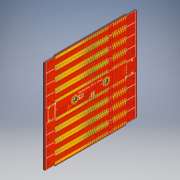
# Autodesk Inventor part: Backplane_PCB
Saved by Autodesk Inventor 2018 (Build 220112000, 112)
## iProperties
Created: 2018-10-18
Part Number: Backplane_PCB
Material: Epoxy Resin
Document SubType Name: Modeling
Designer: Bradley
Density: 1.14 g/cm^3
Appearance: Smooth - Dark Gray
Author: Bradley
Autodesk Inventor part; units mm, degrees
ref_plane "YZ Plane" through (0, 0, 0) normal (1, 0, 0) x (0, 1, 0)
ref_plane "XZ Plane" through (0, 0, 0) normal (0, 1, 0) x (-1, 0, 0)
ref_plane "XY Plane" through (0, 0, 0) normal (0, 0, 1) x (1, 0, 0)
sketch "Sketch1" plane through (0, 0, 0) normal (1, 0, 0) x (0, 1, 0)
  line L0 (-41.4, -43) -> (41.4, -43)
  line L1 (41.4, -43) -> (41.4, 43)
  line L2 (41.4, 43) -> (-41.4, 43)
  line L3 (-41.4, 43) -> (-41.4, -43)
  line L4 (-41.4, -43) -> (41.4, 43) construction
  line L5 (41.4, -43) -> (-41.4, 43) construction
  point P0 (0, 0)
  dimension "d0" = 86
  dimension "d1" = 82.8
  constraints: 12 end point, 2 midpoint, 2 parallel, 1 horizontal, 1 perpendicular
  measures "d0" distance of L2.end L0.start
  measures "d1" distance of L1.end L2.end
extrude "Extrusion1" add sketch "Sketch1" along normal mid plane 1
sketch "Sketch9" plane through (0.5, 0, 0) normal (1, 0, 0) x (0, 0, -1)
  line L0 (43, -41.4) -> (43, 41.4) projected
  line L1 (43, 41.4) -> (-43, 41.4) projected
  line L2 (-43, 41.4) -> (-43, -41.4) projected
  line L3 (-43, -41.4) -> (43, -41.4) projected
  line L4 (45, 36.5) -> (-45, 36.5) construction
  line L5 (-45, 36.5) -> (-45, -36.5) construction
  line L6 (-45, -36.5) -> (45, -36.5) construction
  line L7 (45, -36.5) -> (45, 36.5) construction
  line L8 (45, 36.5) -> (-45, -36.5) construction
  line L9 (-45, 36.5) -> (45, -36.5) construction
  circle A0 centre (-45, -36.5) radius 3 construction
  line L10 (-41.9, -41.4) -> (-41.9, -32)
  line L11 (-41.9, -32) -> (-43, -32)
  line L12 (-43, 41.4) -> (-43, -41.4) projected
  line L13 (-41.9, 41.4) -> (-41.9, 32)
  line L14 (-41.9, 32) -> (-43, 32)
  line L15 (43, 41.4) -> (-43, 41.4) projected
  line L16 (41.9, 41.4) -> (41.9, 32)
  line L17 (41.9, 32) -> (43, 32)
  line L18 (41.9, -41.4) -> (41.9, -32)
  line L19 (41.9, -32) -> (43, -32)
  point P0 (0, 0)
  dimension "d57" = 90
  dimension "d58" = 73
  dimension "d59" = 6
  dimension "d60" = 1.1
  dimension "d61" = 32
  constraints: 28 end point, 8 point on line, 6 collinear, 6 perpendicular, 3 vertical, 2 midpoint, 2 parallel, 1 centre point, 1 coincident, 1 horizontal
  measures "d57" distance of L6.end L5.end
  measures "d58" distance of L5.end L4.end
  measures "d59" diameter of A0
  measures "d60" distance between parallel lines of L10 L2
  measures "d61" distance from line of point (0, 0) L11
extrude "Extrusion2" cut sketch "Sketch9" against normal through all contours L3 L18 L19 L0 | L17 L16 L1 L0 | L3 L2 L11 L10 | L13 L14 L2 L1
fillet "Fillet1" radius 0.5 12 edges at (0, -41.4, -41.9) (0, -32, -41.9) (0, -32, -43) (0, 41.4, -41.9) (0, 32, -41.9) (0, 32, -43) (0, 41.4, 41.9) (0, 32, 43) (0, 32, 41.9) (0, -32, 43) (0, -32, 41.9) (0, -41.4, 41.9)
sketch "Sketch7" plane through (0.5, 0, 0) normal (1, 0, 0) x (0, 0, -1)
  line L0 (43, -31.5) -> (43, 31.5) projected
  line L1 (41.4, 41.4) -> (-41.4, 41.4) projected
  line L2 (-43, 31.5) -> (-43, -31.5) projected
  line L3 (-41.4, -41.4) -> (41.4, -41.4) projected
  line L4 (-43, -41.4) -> (43, -41.4) projected
  line L5 (43, 41.4) -> (-43, 41.4) projected
  arc A0 (-41.9, -40.9) -> (-41.4, -41.4) centre (-41.4, -40.9) ccw projected
  arc A1 (41.4, -41.4) -> (41.9, -40.9) centre (41.4, -40.9) ccw projected
  line L6 (41.9, -40.9) -> (41.9, -32.5) projected
  arc A2 (42.4, -32) -> (41.9, -32.5) centre (42.4, -32.5) ccw projected
  line L7 (42.4, -32) -> (42.5, -32) projected
  arc A3 (42.5, -32) -> (43, -31.5) centre (42.5, -31.5) ccw projected
  arc A4 (43, 31.5) -> (42.5, 32) centre (42.5, 31.5) ccw projected
  line L8 (42.5, 32) -> (42.4, 32) projected
  arc A5 (41.9, 32.5) -> (42.4, 32) centre (42.4, 32.5) ccw projected
  line L9 (41.9, 32.5) -> (41.9, 40.9) projected
  arc A6 (41.9, 40.9) -> (41.4, 41.4) centre (41.4, 40.9) ccw projected
  arc A7 (-41.4, 41.4) -> (-41.9, 40.9) centre (-41.4, 40.9) ccw projected
  line L10 (-41.9, 40.9) -> (-41.9, 32.5) projected
  arc A8 (-42.4, 32) -> (-41.9, 32.5) centre (-42.4, 32.5) ccw projected
  line L11 (-42.4, 32) -> (-42.5, 32) projected
  arc A9 (-42.5, 32) -> (-43, 31.5) centre (-42.5, 31.5) ccw projected
  arc A10 (-43, -31.5) -> (-42.5, -32) centre (-42.5, -31.5) ccw projected
  line L12 (-42.5, -32) -> (-42.4, -32) projected
  arc A11 (-41.9, -32.5) -> (-42.4, -32) centre (-42.4, -32.5) ccw projected
  line L13 (-41.9, -32.5) -> (-41.9, -40.9) projected
  line L14 (-43.0019, -41.4) -> (-43.0019, 41.4) construction
  line L15 (-43.0019, 41.4) -> (43.0019, 41.4) construction
  line L16 (43.0019, 41.4) -> (43.0019, -41.4) construction
  line L17 (43.0019, -41.4) -> (-43.0019, -41.4) construction
  point P0 (0, 0)
  point P1 (0, 41.4)
  point P2 (0, 41.4)
  constraints: 3 midpoint, 2 collinear, 2 other
decal "Decal1"
sketch "Sketch8" plane through (-0.5, 0, 0) normal (-1, 0, 0) x (0, 0, 1)
  line L0 (-43, 31.5) -> (-43, -31.5) projected
  line L1 (-41.4, -41.4) -> (41.4, -41.4) projected
  line L2 (43, -31.5) -> (43, 31.5) projected
  line L3 (41.4, 41.4) -> (-41.4, 41.4) projected
  line L4 (43, 41.4) -> (-43, 41.4) projected
  line L5 (-43, -41.4) -> (43, -41.4) projected
  arc A0 (41.4, -41.4) -> (41.9, -40.9) centre (41.4, -40.9) ccw projected
  line L6 (41.9, -40.9) -> (41.9, -32.5) projected
  arc A1 (42.4, -32) -> (41.9, -32.5) centre (42.4, -32.5) ccw projected
  line L7 (42.4, -32) -> (42.5, -32) projected
  arc A2 (42.5, -32) -> (43, -31.5) centre (42.5, -31.5) ccw projected
  arc A3 (43, 31.5) -> (42.5, 32) centre (42.5, 31.5) ccw projected
  line L8 (42.5, 32) -> (42.4, 32) projected
  arc A4 (41.9, 32.5) -> (42.4, 32) centre (42.4, 32.5) ccw projected
  line L9 (41.9, 32.5) -> (41.9, 40.9) projected
  arc A5 (41.9, 40.9) -> (41.4, 41.4) centre (41.4, 40.9) ccw projected
  arc A6 (-41.4, 41.4) -> (-41.9, 40.9) centre (-41.4, 40.9) ccw projected
  line L10 (-41.9, 40.9) -> (-41.9, 32.5) projected
  arc A7 (-42.4, 32) -> (-41.9, 32.5) centre (-42.4, 32.5) ccw projected
  line L11 (-42.4, 32) -> (-42.5, 32) projected
  arc A8 (-42.5, 32) -> (-43, 31.5) centre (-42.5, 31.5) ccw projected
  arc A9 (-43, -31.5) -> (-42.5, -32) centre (-42.5, -31.5) ccw projected
  line L12 (-42.5, -32) -> (-42.4, -32) projected
  arc A10 (-41.9, -32.5) -> (-42.4, -32) centre (-42.4, -32.5) ccw projected
  line L13 (-41.9, -32.5) -> (-41.9, -40.9) projected
  arc A11 (-41.9, -40.9) -> (-41.4, -41.4) centre (-41.4, -40.9) ccw projected
  line L14 (43.0019, 41.4) -> (43.0019, -41.4) construction
  line L15 (43.0019, -41.4) -> (-43.0019, -41.4) construction
  line L16 (-43.0019, -41.4) -> (-43.0019, 41.4) construction
  line L17 (-43.0019, 41.4) -> (43.0019, 41.4) construction
  point P0 (0, 0)
  point P1 (0, -41.4)
  point P2 (0, -41.4)
  constraints: 3 midpoint, 2 collinear, 2 other
decal "Decal2"
sketch "Sketch2" plane through (0.5, 0, 0) normal (1, 0, 0) x (0, 0, -1)
  line L0 (0, -14) -> (0, 14) construction
  point P0 (0, 0)
  point P1 (0, 0)
  dimension "d7" = 28
  constraints: 3 coincident, 2 end point, 1 midpoint, 1 vertical
  measures "d7" distance of L0.start L0.end
hole "Hole1" at (0.5, -14, 0) at (0.5, 14, 0) direction (-1, 0, 0) diameter 3.3 end through all
sketch "Sketch3" plane through (0.5, 0, 0) normal (1, 0, 0) x (0, 0, -1)
  point P0 (0, 0)
  point P1 (-37.5, 38.3)
  point P2 (-28.5, 38.3)
  point P3 (-19.5, 38.3)
  point P4 (-10.5, 38.3)
  point P5 (10.5, 38.3)
  point P6 (19.5, 38.3)
  point P7 (28.5, 38.3)
  point P8 (37.5, 38.3)
  constraints: 8 other
hole "Hole2" at (0.5, 38.3, 37.5) at (0.5, 38.3, 28.5) at (0.5, 38.3, 19.5) at (0.5, 38.3, 10.5) at (0.5, 38.3, -10.5) at (0.5, 38.3, -19.5) at (0.5, 38.3, -28.5) at (0.5, 38.3, -37.5) direction (-1, 0, 0) diameter 1.05 end through all
sketch "Sketch4" plane through (0.5, 0, 0) normal (1, 0, 0) x (0, 0, -1)
  point P0 (0, 0)
  point P1 (-37.5, -38.3)
  point P2 (-28.5, -38.3)
  point P3 (-19.5, -38.3)
  point P4 (-10.5, -38.3)
  point P5 (10.5, -38.3)
  point P6 (19.5, -38.3)
  point P7 (28.5, -38.3)
  point P8 (37.5, -38.3)
  constraints: 8 other
hole "Hole3" at (0.5, -38.3, 37.5) at (0.5, -38.3, 28.5) at (0.5, -38.3, 19.5) at (0.5, -38.3, 10.5) at (0.5, -38.3, -10.5) at (0.5, -38.3, -19.5) at (0.5, -38.3, -28.5) at (0.5, -38.3, -37.5) direction (-1, 0, 0) diameter 1.45 end through all
sketch "Sketch5" plane through (0.5, 0, 0) normal (1, 0, 0) x (0, 0, -1)
  point P0 (0, 0)
  point P1 (0, -16.3)
  point P2 (0, -11.7)
  point P3 (1.626, -12.374)
  point P4 (2.3, -14)
  point P5 (1.626, -15.626)
  point P6 (-2.3, -14)
  point P7 (-1.626, -15.626)
  point P8 (-1.626, -12.374)
  point P9 (-1.626, 15.626)
  point P10 (0, 11.7)
  point P11 (0, 16.3)
  point P12 (1.626, 15.626)
  point P13 (2.3, 14)
  point P14 (1.626, 12.374)
  point P15 (-2.3, 14)
  point P16 (-1.626, 12.374)
  constraints: 16 other
hole "Hole4" at (0.5, -16.3, 0) at (0.5, -11.7, 0) at (0.5, -12.374, -1.626) at (0.5, -14, -2.3) at (0.5, -15.626, -1.626) at (0.5, -14, 2.3) at (0.5, -15.626, 1.626) at (0.5, -12.374, 1.626) at (0.5, 15.626, 1.626) at (0.5, 11.7, 0) at (0.5, 16.3, 0) at (0.5, 15.626, -1.626) at (0.5, 14, -2.3) at (0.5, 12.374, -1.626) at (0.5, 14, 2.3) at (0.5, 12.374, 1.626) direction (-1, 0, 0) diameter 0.45 end through all
sketch "Sketch10" plane through (0.5, 0, 0) normal (1, 0, 0) x (0, 0, -1)
  point P0 (0, 0)
  point P1 (17.575, -9.45)
  point P2 (8.575, -9.45)
  point P3 (-12.425, -9.45)
  point P4 (-21.425, -9.45)
  point P5 (-30.425, -9.45)
  point P6 (-39.425, -9.45)
  point P7 (35.575, -10.65)
  point P8 (26.575, -10.65)
  point P9 (17.575, -10.65)
  point P10 (8.575, -10.65)
  point P11 (-12.425, -10.65)
  point P12 (-21.425, -10.65)
  point P13 (-30.425, -10.65)
  point P14 (-39.425, -10.65)
  point P15 (35.575, -16.65)
  point P16 (26.575, -16.65)
  point P17 (17.575, -16.65)
  point P18 (8.575, -16.65)
  point P19 (-12.425, -16.65)
  point P20 (-21.425, -16.65)
  point P21 (-30.425, -16.65)
  point P22 (-39.425, -16.65)
  point P23 (35.575, -17.85)
  point P24 (26.575, -17.85)
  point P25 (17.575, -17.85)
  point P26 (8.575, -17.85)
  point P27 (-12.425, -17.85)
  point P28 (-21.425, -17.85)
  point P29 (-30.425, -17.85)
  point P30 (-39.425, -17.85)
  point P31 (35.575, -19.05)
  point P32 (26.575, -19.05)
  point P33 (17.575, -19.05)
  point P34 (8.575, -19.05)
  point P35 (-12.425, -19.05)
  point P36 (-21.425, -19.05)
  point P37 (-30.425, -19.05)
  point P38 (-39.425, -19.05)
  point P39 (35.575, -21.45)
  point P40 (26.575, -21.45)
  point P41 (17.575, -21.45)
  point P42 (8.575, -21.45)
  point P43 (-12.425, -21.45)
  point P44 (-21.425, -21.45)
  point P45 (-30.425, -21.45)
  point P46 (-39.425, -21.45)
  point P47 (35.575, -22.65)
  point P48 (26.575, -22.65)
  point P49 (17.575, -22.65)
  point P50 (8.575, -22.65)
  point P51 (-12.425, -22.65)
  point P52 (-21.425, -22.65)
  point P53 (-30.425, -22.65)
  point P54 (-39.425, -22.65)
  point P55 (35.575, -11.85)
  point P56 (26.575, -11.85)
  point P57 (17.575, -11.85)
  point P58 (8.575, -11.85)
  point P59 (-12.425, -11.85)
  point P60 (-21.425, -11.85)
  point P61 (-30.425, -11.85)
  point P62 (-39.425, -11.85)
  point P63 (35.575, -13.05)
  point P64 (26.575, -13.05)
  point P65 (17.575, -13.05)
  point P66 (8.575, -13.05)
  point P67 (-12.425, -13.05)
  point P68 (-21.425, -13.05)
  point P69 (-30.425, -13.05)
  point P70 (-39.425, -13.05)
  point P71 (35.575, -14.25)
  point P72 (26.575, -14.25)
  point P73 (17.575, -14.25)
  point P74 (8.575, -14.25)
  point P75 (-12.425, -14.25)
  point P76 (-21.425, -14.25)
  point P77 (-30.425, -14.25)
  point P78 (-39.425, -14.25)
  point P79 (35.575, -15.45)
  point P80 (26.575, -15.45)
  point P81 (17.575, -15.45)
  point P82 (8.575, -15.45)
  point P83 (-12.425, -15.45)
  point P84 (-21.425, -15.45)
  point P85 (-30.425, -15.45)
  point P86 (-39.425, -15.45)
  point P87 (35.575, 3.75)
  point P88 (26.575, 3.75)
  point P89 (17.575, 3.75)
  point P90 (8.575, 3.75)
  point P91 (-12.425, 3.75)
  point P92 (-21.425, 3.75)
  point P93 (-30.425, 3.75)
  point P94 (-39.425, 3.75)
  point P95 (35.575, 2.55)
  point P96 (26.575, 2.55)
  point P97 (17.575, 2.55)
  point P98 (8.575, 2.55)
  point P99 (-12.425, 2.55)
  point P100 (-21.425, 2.55)
  point P101 (-30.425, 2.55)
  point P102 (-39.425, 2.55)
  point P103 (35.575, 1.35)
  point P104 (26.575, 1.35)
  point P105 (17.575, 1.35)
  point P106 (8.575, 1.35)
  point P107 (-12.425, 1.35)
  point P108 (-21.425, 1.35)
  point P109 (-30.425, 1.35)
  point P110 (-39.425, 1.35)
  point P111 (35.575, -1.05)
  point P112 (26.575, -1.05)
  point P113 (17.575, -1.05)
  point P114 (8.575, -1.05)
  point P115 (-12.425, -1.05)
  point P116 (-21.425, -1.05)
  point P117 (-30.425, -1.05)
  point P118 (-39.425, -1.05)
  point P119 (35.575, -2.25)
  point P120 (26.575, -2.25)
  point P121 (17.575, -2.25)
  point P122 (8.575, -2.25)
  point P123 (-12.425, -2.25)
  point P124 (-21.425, -2.25)
  point P125 (-30.425, -2.25)
  point P126 (-39.425, -2.25)
  point P127 (35.575, -3.45)
  point P128 (26.575, -3.45)
  point P129 (17.575, -3.45)
  point P130 (8.575, -3.45)
  point P131 (-12.425, -3.45)
  point P132 (-21.425, -3.45)
  point P133 (-30.425, -3.45)
  point P134 (-39.425, -3.45)
  point P135 (35.575, -4.65)
  point P136 (26.575, -4.65)
  point P137 (17.575, -4.65)
  point P138 (8.575, -4.65)
  point P139 (-12.425, -4.65)
  point P140 (-21.425, -4.65)
  point P141 (-30.425, -4.65)
  point P142 (-39.425, -4.65)
  point P143 (35.575, -5.85)
  point P144 (26.575, -5.85)
  point P145 (17.575, -5.85)
  point P146 (8.575, -5.85)
  point P147 (-12.425, -5.85)
  point P148 (-21.425, -5.85)
  point P149 (-30.425, -5.85)
  point P150 (-39.425, -5.85)
  point P151 (35.575, -7.05)
  point P152 (26.575, -7.05)
  point P153 (17.575, -7.05)
  point P154 (8.575, -7.05)
  point P155 (-12.425, -7.05)
  point P156 (-21.425, -7.05)
  point P157 (-30.425, -7.05)
  point P158 (-39.425, -7.05)
  point P159 (35.575, -27.45)
  point P160 (26.575, -27.45)
  point P161 (17.575, -27.45)
  point P162 (8.575, -27.45)
  point P163 (-12.425, -27.45)
  point P164 (-21.425, -27.45)
  point P165 (-30.425, -27.45)
  point P166 (-39.425, -27.45)
  point P167 (35.575, -28.65)
  point P168 (26.575, -28.65)
  point P169 (17.575, -28.65)
  point P170 (8.575, -28.65)
  point P171 (-12.425, -28.65)
  point P172 (-21.425, -28.65)
  point P173 (-30.425, -28.65)
  point P174 (-39.425, -28.65)
  point P175 (35.575, -29.85)
  point P176 (26.575, -29.85)
  point P177 (17.575, -29.85)
  point P178 (8.575, -29.85)
  point P179 (-12.425, -29.85)
  point P180 (-21.425, -29.85)
  point P181 (-30.425, -29.85)
  point P182 (-39.425, -29.85)
  point P183 (35.575, -31.05)
  point P184 (26.575, -31.05)
  point P185 (17.575, -31.05)
  point P186 (8.575, -31.05)
  point P187 (-12.425, -31.05)
  point P188 (-21.425, -31.05)
  point P189 (-30.425, -31.05)
  point P190 (-39.425, -31.05)
  point P191 (39.425, -27.75)
  point P192 (30.425, -27.75)
  point P193 (-35.575, -27.75)
  point P194 (-26.575, -27.75)
  point P195 (-17.575, -27.75)
  point P196 (-8.575, -27.75)
  point P197 (12.425, -27.75)
  point P198 (21.425, -27.75)
  point P199 (39.425, -28.95)
  constraints: 284 other
hole "Hole6" at (0.5, -9.45, -17.575) at (0.5, -9.45, -8.575) at (0.5, -9.45, 12.425) at (0.5, -9.45, 21.425) at (0.5, -9.45, 30.425) at (0.5, -9.45, 39.425) at (0.5, -10.65, -35.575) at (0.5, -10.65, -26.575) at (0.5, -10.65, -17.575) at (0.5, -10.65, -8.575) at (0.5, -10.65, 12.425) at (0.5, -10.65, 21.425) at (0.5, -10.65, 30.425) at (0.5, -10.65, 39.425) at (0.5, -16.65, -35.575) at (0.5, -16.65, -26.575) at (0.5, -16.65, -17.575) at (0.5, -16.65, -8.575) at (0.5, -16.65, 12.425) at (0.5, -16.65, 21.425) at (0.5, -16.65, 30.425) at (0.5, -16.65, 39.425) at (0.5, -17.85, -35.575) at (0.5, -17.85, -26.575) at (0.5, -17.85, -17.575) at (0.5, -17.85, -8.575) at (0.5, -17.85, 12.425) at (0.5, -17.85, 21.425) at (0.5, -17.85, 30.425) at (0.5, -17.85, 39.425) at (0.5, -19.05, -35.575) at (0.5, -19.05, -26.575) at (0.5, -19.05, -17.575) at (0.5, -19.05, -8.575) at (0.5, -19.05, 12.425) at (0.5, -19.05, 21.425) at (0.5, -19.05, 30.425) at (0.5, -19.05, 39.425) at (0.5, -21.45, -35.575) at (0.5, -21.45, -26.575) at (0.5, -21.45, -17.575) at (0.5, -21.45, -8.575) at (0.5, -21.45, 12.425) at (0.5, -21.45, 21.425) at (0.5, -21.45, 30.425) at (0.5, -21.45, 39.425) at (0.5, -22.65, -35.575) at (0.5, -22.65, -26.575) at (0.5, -22.65, -17.575) at (0.5, -22.65, -8.575) direction (-1, 0, 0) diameter 0.3 end through all and at (0.5, -22.65, 12.425) (0.5, -22.65, 21.425) (0.5, -22.65, 30.425) (0.5, -22.65, 39.425) (0.5, -11.85, -35.575) (0.5, -11.85, -26.575) (0.5, -11.85, -17.575) (0.5, -11.85, -8.575) (0.5, -11.85, 12.425) (0.5, -11.85, 21.425) (0.5, -11.85, 30.425) (0.5, -11.85, 39.425) (0.5, -13.05, -35.575) (0.5, -13.05, -26.575) (0.5, -13.05, -17.575) (0.5, -13.05, -8.575) (0.5, -13.05, 12.425) (0.5, -13.05, 21.425) (0.5, -13.05, 30.425) (0.5, -13.05, 39.425) (0.5, -14.25, -35.575) (0.5, -14.25, -26.575) (0.5, -14.25, -17.575) (0.5, -14.25, -8.575) (0.5, -14.25, 12.425) (0.5, -14.25, 21.425) (0.5, -14.25, 30.425) (0.5, -14.25, 39.425) (0.5, -15.45, -35.575) (0.5, -15.45, -26.575) (0.5, -15.45, -17.575) (0.5, -15.45, -8.575) (0.5, -15.45, 12.425) (0.5, -15.45, 21.425) (0.5, -15.45, 30.425) (0.5, -15.45, 39.425) (0.5, 3.75, -35.575) (0.5, 3.75, -26.575) (0.5, 3.75, -17.575) (0.5, 3.75, -8.575) (0.5, 3.75, 12.425) (0.5, 3.75, 21.425) (0.5, 3.75, 30.425) (0.5, 3.75, 39.425) (0.5, 2.55, -35.575) (0.5, 2.55, -26.575) (0.5, 2.55, -17.575) (0.5, 2.55, -8.575) (0.5, 2.55, 12.425) (0.5, 2.55, 21.425) (0.5, 2.55, 30.425) (0.5, 2.55, 39.425) (0.5, 1.35, -35.575) (0.5, 1.35, -26.575) (0.5, 1.35, -17.575) (0.5, 1.35, -8.575) (0.5, 1.35, 12.425) (0.5, 1.35, 21.425) (0.5, 1.35, 30.425) (0.5, 1.35, 39.425) (0.5, -1.05, -35.575) (0.5, -1.05, -26.575) (0.5, -1.05, -17.575) (0.5, -1.05, -8.575) (0.5, -1.05, 12.425) (0.5, -1.05, 21.425) (0.5, -1.05, 30.425) (0.5, -1.05, 39.425) (0.5, -2.25, -35.575) (0.5, -2.25, -26.575) (0.5, -2.25, -17.575) (0.5, -2.25, -8.575) (0.5, -2.25, 12.425) (0.5, -2.25, 21.425) (0.5, -2.25, 30.425) (0.5, -2.25, 39.425) (0.5, -3.45, -35.575) (0.5, -3.45, -26.575) (0.5, -3.45, -17.575) (0.5, -3.45, -8.575) (0.5, -3.45, 12.425) (0.5, -3.45, 21.425) (0.5, -3.45, 30.425) (0.5, -3.45, 39.425) (0.5, -4.65, -35.575) (0.5, -4.65, -26.575) (0.5, -4.65, -17.575) (0.5, -4.65, -8.575) (0.5, -4.65, 12.425) (0.5, -4.65, 21.425) (0.5, -4.65, 30.425) (0.5, -4.65, 39.425) (0.5, -5.85, -35.575) (0.5, -5.85, -26.575) (0.5, -5.85, -17.575) (0.5, -5.85, -8.575) (0.5, -5.85, 12.425) (0.5, -5.85, 21.425) (0.5, -5.85, 30.425) (0.5, -5.85, 39.425) (0.5, -7.05, -35.575) (0.5, -7.05, -26.575) (0.5, -7.05, -17.575) (0.5, -7.05, -8.575) (0.5, -7.05, 12.425) (0.5, -7.05, 21.425) (0.5, -7.05, 30.425) (0.5, -7.05, 39.425) (0.5, -27.45, -35.575) (0.5, -27.45, -26.575) (0.5, -27.45, -17.575) (0.5, -27.45, -8.575) (0.5, -27.45, 12.425) (0.5, -27.45, 21.425) (0.5, -27.45, 30.425) (0.5, -27.45, 39.425) (0.5, -28.65, -35.575) (0.5, -28.65, -26.575) (0.5, -28.65, -17.575) (0.5, -28.65, -8.575) (0.5, -28.65, 12.425) (0.5, -28.65, 21.425) (0.5, -28.65, 30.425) (0.5, -28.65, 39.425) (0.5, -29.85, -35.575) (0.5, -29.85, -26.575) (0.5, -29.85, -17.575) (0.5, -29.85, -8.575) (0.5, -29.85, 12.425) (0.5, -29.85, 21.425) (0.5, -29.85, 30.425) (0.5, -29.85, 39.425) (0.5, -31.05, -35.575) (0.5, -31.05, -26.575) (0.5, -31.05, -17.575) (0.5, -31.05, -8.575) (0.5, -31.05, 12.425) (0.5, -31.05, 21.425) (0.5, -31.05, 30.425) (0.5, -31.05, 39.425) (0.5, -27.75, -39.425) (0.5, -27.75, -30.425) (0.5, -27.75, 35.575) (0.5, -27.75, 26.575) (0.5, -27.75, 17.575) (0.5, -27.75, 8.575) (0.5, -27.75, -12.425) (0.5, -27.75, -21.425) (0.5, -28.95, -39.425) (0.5, -28.95, -30.425) (0.5, -28.95, -21.425) (0.5, -28.95, -12.425) (0.5, -28.95, 8.575) (0.5, -28.95, 17.575) (0.5, -23.85, -35.575) (0.5, -28.95, 35.575) (0.5, -30.15, -39.425) (0.5, -30.15, -30.425) (0.5, -30.15, -21.425) (0.5, -30.15, -12.425) (0.5, -30.15, 35.575) (0.5, -30.15, 26.575) (0.5, -30.15, 17.575) (0.5, -30.15, 8.575) (0.5, -31.35, -39.425) (0.5, -31.35, -30.425) (0.5, -31.35, -21.425) (0.5, -31.35, -12.425) (0.5, -31.35, 8.575) (0.5, -31.35, 17.575) (0.5, -31.35, 26.575) (0.5, -31.35, 35.575) (0.5, 32.3, 1.5) (0.5, 4, -0.4) (0.5, -20.25, -35.575) (0.5, -20.25, -26.575) (0.5, -20.25, -17.575) (0.5, -20.25, -8.575) (0.5, -20.25, 12.425) (0.5, -20.25, 21.425) (0.5, -20.25, 30.425) (0.5, -20.25, 39.425) (0.5, 4, -5.7) (0.5, 32.3, -1.5) (0.5, 13.05, 5.8) (0.5, 13.65, -4.25) (0.5, 12.15, -5.8) (0.5, 11.85, 5.8) (0.5, 10.95, -5.8) (0.5, 10.65, 5.8) (0.5, 4, -4.9) (0.5, 0.15, -8.575) (0.5, 0.15, -35.575) (0.5, -28.95, 26.575) (0.5, 0.15, -17.575) (0.5, 0.15, 12.425) (0.5, 0.15, 21.425) (0.5, 0.15, 30.425) (0.5, 0.15, 39.425) (0.5, -23.85, -26.575) (0.5, -23.85, -17.575) (0.5, -23.85, -8.575) (0.5, -23.85, 12.425) (0.5, -23.85, 21.425) (0.5, -23.85, 30.425) (0.5, -23.85, 39.425) (0.5, -25.05, -35.575) (0.5, -25.05, -26.575) (0.5, -25.05, -17.575) (0.5, -25.05, -8.575) (0.5, -25.05, 12.425) (0.5, -25.05, 21.425) (0.5, -25.05, 30.425) (0.5, -25.05, 39.425) (0.5, -26.25, -35.575) (0.5, -26.25, -26.575) (0.5, -26.25, -17.575) (0.5, -26.25, -8.575) (0.5, -26.25, 12.425) (0.5, -26.25, 21.425) (0.5, -26.25, 30.425) (0.5, -26.25, 39.425) (0.5, -8.25, -35.575) (0.5, -8.25, -26.575) (0.5, -8.25, -17.575) (0.5, -8.25, -8.575) (0.5, -8.25, 12.425) (0.5, -8.25, 21.425) (0.5, -8.25, 30.425) (0.5, -8.25, 39.425) (0.5, -9.45, -35.575) (0.5, -9.45, -26.575) (0.5, 0.15, -26.575)
body "Solid1"
